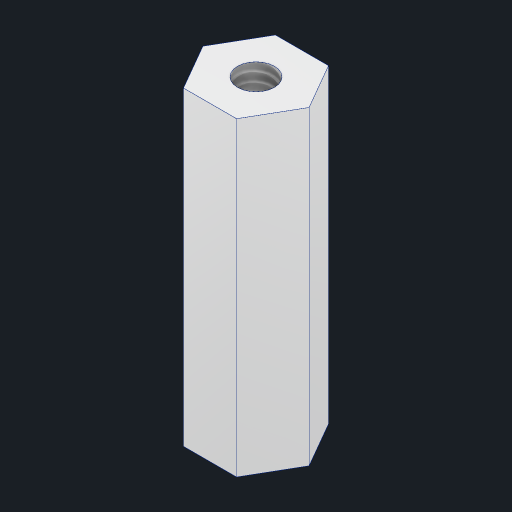
# Autodesk Inventor part: OUTK_016_Shaft4
Saved by Autodesk Inventor 2024.2 (Build 282272000, 272)
## iProperties
Created: 2024-12-08
Part Number: OUTK_016_Shaft4
Material: Aluminum 6061
Document SubType Name: Modeling
Designer: Bryan
Density: 2.7 g/cm^3
Appearance: Aluminum - Flat
Author: Bryan
Autodesk Inventor part; units mm, degrees
ref_plane "YZ Plane" through (0, 0, 0) normal (1, 0, 0) x (0, 1, 0)
ref_plane "XZ Plane" through (0, 0, 0) normal (0, 1, 0) x (-1, 0, 0)
ref_plane "XY Plane" through (0, 0, 0) normal (0, 0, 1) x (1, 0, 0)
sketch "Sketch1" plane through (0, 0, 0) normal (0, 1, 0) x (-1, 0, 0)
  line L0 (-3.6662, 6.35) -> (3.6662, 6.35)
  line L1 (3.6662, 6.35) -> (7.3323, 0)
  line L2 (7.3323, 0) -> (3.6662, -6.35)
  line L3 (3.6662, -6.35) -> (-3.6662, -6.35)
  line L4 (-3.6662, -6.35) -> (-7.3323, 0)
  line L5 (-7.3323, 0) -> (-3.6662, 6.35)
  point P0 (0, 0)
  point P1 (0, 0)
  dimension "d0" = 12.7
  constraints: 12 end point, 1 coincident, 1 horizontal, 13 other
  measures "d0" distance between parallel lines of L3 L0
extrude "Extrusion1" add sketch "Sketch1" along normal blind 42.8625
sketch "Sketch2" plane through (0, 42.8625, 0) normal (0, 1, 0) x (1, 0, 0)
  circle A0 centre (0, 0) radius 2.54
  dimension "d3" = 5.08
  constraints: 1 centre point, 1 coincident
  measures "d3" diameter of A0
extrude "Extrusion2" cut sketch "Sketch2" against normal blind 25.4
thread "Thread1" size "1/4-20 UNC" class "2B" standard "ANSI Unified Screw Threads" full length
sketch "Sketch3" plane through (0, 0, 0) normal (0, -1, 0) x (1, 0, 0)
  circle A0 centre (0, 0) radius 2.54
  dimension "d8" = 5.08
  constraints: 1 centre point, 1 coincident
  measures "d8" diameter of A0
extrude "Extrusion3" cut sketch "Sketch3" against normal blind 25.4
thread "Thread2" size "1/4-20 UNC" class "2B" standard "ANSI Unified Screw Threads" full length
body "Solid1"
